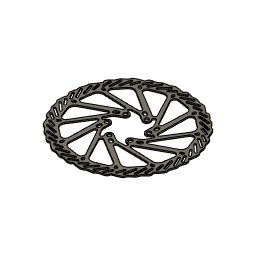
67part (Autodesk Fusion 360 design; units mm, degrees)
Autodesk Fusion 360 part; units mm, degrees
(part 1 of 2)
sketch "Sketch1" plane through (0, 0, 0) normal (0, 1, 0) x (1, 0, 0)
  circle A0 centre (0, 0) radius 80
  circle A1 centre (0, 0) radius 21.9
  dimension "d1" = 160
  dimension "d2" = 43.8
  constraint coincident A0.centre A1.centre
  constraint concentric A0 A1
  measures "d1" diameter of A0
  measures "d2" diameter of A1
sketch "Sketch2" plane through (0, 0, 0) normal (0, 1, 0) x (1, 0, 0)
  spline S0 degree 3 poles (-63.4968, -44.9071) (-64.7262, -42.3768) (-65.0842, -41.971) (-67.4116, -40.491) knots 0 0 0 0 1 1 1 1
  spline S1 degree 3 poles (-67.4116, -40.491) (-69.3332, -39.2736) (-69.9539, -38.6649) (-70.3239, -37.6862) knots 0 0 0 0 1 1 1 1
  spline S2 degree 3 poles (-70.3239, -37.6862) (-70.5984, -36.9224) (-71.5174, -33.3417) (-71.5174, -32.9956) knots 0 0 0 0 1 1 1 1
  spline S3 degree 3 poles (-71.5174, -32.9956) (-71.5174, -32.3869) (-72.1619, -31.1576) (-72.89, -30.3579) knots 0 0 0 0 1 1 1 1
  spline S4 degree 3 poles (-72.89, -30.3579) (-73.7613, -29.4269) (-74.1909, -28.7227) (-74.4416, -27.8873) knots 0 0 0 0 1 1 1 1
  spline S5 degree 3 poles (-74.4416, -27.8873) (-74.6325, -27.2547) (-75.0025, -24.8437) (-75.2174, -22.8625) knots 0 0 0 0 1 1 1 1
  spline S6 degree 3 poles (-75.2174, -22.8625) (-75.3725, -21.4541) (-75.5754, -20.917) (-76.3154, -19.9144) knots 0 0 0 0 1 1 1 1
  spline S7 degree 3 poles (-76.3154, -19.9144) (-77.2464, -18.6851) (-77.4254, -18.1122) (-77.4015, -16.5128) knots 0 0 0 0 1 1 1 1
  spline S8 degree 3 poles (-77.4015, -16.5128) (-77.3777, -14.818) (-77.1986, -11.2254) (-76.9361, -7.2032) knots 0 0 0 0 1 1 1 1
  spline S9 degree 3 poles (-76.9361, -7.2032) (-76.7809, -4.8639) (-76.769, -4.0165) (-76.8645, -3.5271) knots 0 0 0 0 1 1 1 1
  spline S10 degree 3 poles (-76.8645, -3.5271) (-76.9361, -3.181) (-77.497, -1.892) (-78.1057, -0.6626) knots 0 0 0 0 1 1 1 1
  line L0 (-78.1057, -0.6626) -> (-79.2157, 1.5574)
  line L1 (-79.2157, 1.5574) -> (-79.1919, 2.7628)
  spline S11 degree 3 poles (-79.1919, 2.7628) (-79.1799, 4.0041) (-78.9293, 5.0903) (-77.9625, 8.1815) knots 0 0 0 0 1 1 1 1
  line L2 (-77.9625, 8.1815) -> (-77.5686, 9.4109)
  line L3 (-77.5686, 9.4109) -> (-77.7954, 10.4492)
  spline S12 degree 3 poles (-77.7954, 10.4492) (-77.9386, 11.0818) (-78.0222, 11.9412) (-78.0222, 12.6692) knots 0 0 0 0 1 1 1 1
  spline S13 degree 3 poles (-78.0222, 12.6692) (-78.0222, 14.0537) (-77.7357, 15.0444) (-76.4945, 17.9208) knots 0 0 0 0 1 1 1 1
  spline S14 degree 3 poles (-76.4945, 17.9208) (-75.6351, 19.926) (-75.5516, 20.3318) (-75.7306, 21.7759) knots 0 0 0 0 1 1 1 1
  spline S15 degree 3 poles (-75.7306, 21.7759) (-75.9454, 23.5662) (-75.838, 23.8527) (-73.4271, 27.6959) knots 0 0 0 0 1 1 1 1
  spline S16 degree 3 poles (-73.4271, 27.6959) (-72.3051, 29.4743) (-70.9684, 31.5749) (-70.4432, 32.3626) knots 0 0 0 0 1 1 1 1
  spline S17 degree 3 poles (-70.4432, 32.3626) (-69.011, 34.5349) (-68.4858, 35.4062) (-68.2352, 36.0029) knots 0 0 0 0 1 1 1 1
  spline S18 degree 3 poles (-68.2352, 36.0029) (-68.0681, 36.4207) (-67.9845, 37.1368) (-67.8771, 39.13) knots 0 0 0 0 1 1 1 1
  spline S19 degree 3 poles (-67.8771, 39.13) (-67.7458, 41.7081) (-67.7339, 41.72) (-67.34, 42.5077) knots 0 0 0 0 1 1 1 1
  spline S20 degree 3 poles (-67.34, 42.5077) (-67.0058, 43.1522) (-66.5284, 43.7132) (-64.8216, 45.42) knots 0 0 0 0 1 1 1 1
  spline S21 degree 3 poles (-20.3623, 43.2597) (15.6024, 24.417) (-7.9458, 24.9808) (-14.8839, 23.5424) knots 0 0 0 0 1 1 1 1
  spline S22 degree 3 poles (-14.8839, 23.5424) (-16.6504, 23.1724) (-18.3213, 22.8143) (-18.5839, 22.7427) knots 0 0 0 0 1 1 1 1
  spline S23 degree 3 poles (-18.5839, 22.7427) (-20.0042, 22.3369) (-20.78, 20.9524) (-20.2549, 19.735) knots 0 0 0 0 1 1 1 1
  spline S24 degree 3 poles (-20.2549, 19.735) (-19.7894, 18.6608) (-19.2523, 18.3863) (-17.0562, 18.0521) knots 0 0 0 0 1 1 1 1
  spline S25 degree 3 poles (-17.0562, 18.0521) (-16.2446, 17.9327) (-15.6478, 17.7656) (-15.1226, 17.515) knots 0 0 0 0 1 1 1 1
  spline S26 degree 3 poles (-15.1226, 17.515) (-12.3775, 16.1544) (-11.7091, 12.3947) (-13.8097, 10.0076) knots 0 0 0 0 1 1 1 1
  spline S27 degree 3 poles (-13.8097, 10.0076) (-14.5617, 9.1602) (-14.8004, 9.0289) (-17.9275, 7.6683) knots 0 0 0 0 1 1 1 1
  spline S28 degree 3 poles (-17.9275, 7.6683) (-20.7203, 6.4509) (-21.7945, 5.9377) (-22.4032, 5.5199) knots 0 0 0 0 1 1 1 1
  spline S29 degree 3 poles (-22.4032, 5.5199) (-23.0835, 5.0664) (-23.9906, 4.1951) (-24.5516, 3.479) knots 0 0 0 0 1 1 1 1
  spline S30 degree 3 poles (-24.5516, 3.479) (-25.0648, 2.8225) (-25.7332, 1.6767) (-25.6616, 1.5932) knots 0 0 0 0 1 1 1 1
  spline S31 degree 3 poles (-25.6616, 1.5932) (-25.6377, 1.5693) (-25.7213, 1.4141) (-25.8287, 1.2471) knots 0 0 0 0 1 1 1 1
  spline S32 degree 3 poles (-25.8287, 1.2471) (-26.0316, 0.9487) (-27.4996, -3.3839) (-27.9054, -4.8519) knots 0 0 0 0 1 1 1 1
  spline S33 degree 3 poles (-27.9054, -4.8519) (-28.0248, -5.2577) (-28.168, -5.6277) (-28.2396, -5.6755) knots 0 0 0 0 1 1 1 1
  spline S34 degree 3 poles (-28.2396, -5.6755) (-28.3232, -5.7232) (-28.3113, -5.8545) (-28.2038, -6.0455) knots 0 0 0 0 1 1 1 1
  spline S35 degree 3 poles (-28.2038, -6.0455) (-28.1203, -6.2126) (-28.0606, -6.5587) (-28.0964, -6.8332) knots 0 0 0 0 1 1 1 1
  spline S36 degree 3 poles (-28.0964, -6.8332) (-28.1203, -7.1674) (-28.0964, -7.3226) (-27.989, -7.3226) knots 0 0 0 0 1 1 1 1
  spline S37 degree 3 poles (-27.989, -7.3226) (-27.9054, -7.3226) (-27.7861, -7.418) (-27.7264, -7.5493) knots 0 0 0 0 1 1 1 1
  spline S38 degree 3 poles (-27.7264, -7.5493) (-27.5355, -7.8835) (-26.4732, -8.3967) (-25.948, -8.3967) knots 0 0 0 0 1 1 1 1
  spline S39 degree 3 poles (-25.948, -8.3967) (-24.9216, -8.3967) (-24.4681, -8.0984) (-23.4655, -6.7735) knots 0 0 0 0 1 1 1 1
  spline S40 degree 3 poles (-23.4655, -6.7735) (-22.6181, -5.6516) (-21.8781, -4.9832) (-21.0545, -4.6013) knots 0 0 0 0 1 1 1 1
  spline S41 degree 3 poles (-21.0545, -4.6013) (-20.4578, -4.3148) (-20.231, -4.279) (-19.121, -4.279) knots 0 0 0 0 1 1 1 1
  spline S42 degree 3 poles (-19.121, -4.279) (-17.9394, -4.279) (-17.8081, -4.3029) (-17.0681, -4.6729) knots 0 0 0 0 1 1 1 1
  spline S43 degree 3 poles (-17.0681, -4.6729) (-16.161, -5.1145) (-15.242, -6.0335) (-14.8362, -6.8929) knots 0 0 0 0 1 1 1 1
  spline S44 degree 3 poles (-14.8362, -6.8929) (-14.2872, -8.0745) (-14.2752, -8.7548) (-14.693, -12.1564) knots 0 0 0 0 1 1 1 1
  line L4 (-15.1107, -13.3977) -> (-15.0391, -12.6099)
  line L5 (-15.0391, -12.6099) -> (-15.4091, -12.4787)
  spline S45 degree 3 poles (-15.4091, -12.4787) (-15.612, -12.407) (-15.7791, -12.2638) (-15.7791, -12.1683) knots 0 0 0 0 1 1 1 1
  spline S46 degree 3 poles (-15.7791, -12.1683) (-15.7791, -12.049) (-15.7075, -12.0132) (-15.5762, -12.0609) knots 0 0 0 0 1 1 1 1
  spline S47 degree 3 poles (-15.5762, -12.0609) (-15.4449, -12.1087) (-15.4091, -12.0967) (-15.4688, -12.0012) knots 0 0 0 0 1 1 1 1
  spline S48 degree 3 poles (-15.4688, -12.0012) (-15.5165, -11.9177) (-15.4926, -11.858) (-15.433, -11.858) knots 0 0 0 0 1 1 1 1
  spline S49 degree 3 poles (-15.433, -11.858) (-15.3613, -11.858) (-15.3017, -11.8103) (-15.3017, -11.7387) knots 0 0 0 0 1 1 1 1
  spline S50 degree 3 poles (-15.3017, -11.7387) (-15.3017, -11.679) (-15.4091, -11.6193) (-15.5284, -11.6193) knots 0 0 0 0 1 1 1 1
  spline S51 degree 3 poles (-15.5284, -11.6193) (-15.7313, -11.6193) (-15.7433, -11.5716) (-15.6597, -11.2493) knots 0 0 0 0 1 1 1 1
  spline S52 degree 3 poles (-15.6597, -11.2493) (-15.6001, -11.0345) (-15.5762, -10.8196) (-15.612, -10.7719) knots 0 0 0 0 1 1 1 1
  spline S53 degree 3 poles (-15.612, -10.7719) (-15.6478, -10.7122) (-15.6001, -10.6645) (-15.5046, -10.6645) knots 0 0 0 0 1 1 1 1
  spline S54 degree 3 poles (-15.5046, -10.6645) (-15.3255, -10.6645) (-15.1226, -10.9867) (-15.1704, -11.1777) knots 0 0 0 0 1 1 1 1
  spline S55 degree 3 poles (-15.1704, -11.1777) (-15.1823, -11.2374) (-15.1346, -11.2612) (-15.063, -11.2374) knots 0 0 0 0 1 1 1 1
  spline S56 degree 3 poles (-15.063, -11.2374) (-14.9794, -11.2135) (-14.9317, -11.1538) (-14.9436, -11.0941) knots 0 0 0 0 1 1 1 1
  spline S57 degree 3 poles (-14.9436, -11.0941) (-14.9555, -11.0345) (-14.9078, -10.9509) (-14.8362, -10.9032) knots 0 0 0 0 1 1 1 1
  spline S58 degree 3 poles (-14.8362, -10.9032) (-14.5975, -10.76) (-14.8123, -10.4496) (-15.0988, -10.5213) knots 0 0 0 0 1 1 1 1
  line L6 (-15.0988, -10.5213) -> (-15.3613, -10.5809)
  line L7 (-15.3613, -10.5809) -> (-15.1226, -10.3183)
  spline S59 degree 3 poles (-15.1226, -10.3183) (-14.9317, -10.0916) (-14.8839, -9.8648) (-14.872, -9.0055) knots 0 0 0 0 1 1 1 1
  spline S60 degree 3 poles (-14.872, -9.0055) (-14.8601, -8.4445) (-14.8959, -7.9313) (-14.9317, -7.8597) knots 0 0 0 0 1 1 1 1
  spline S61 degree 3 poles (-14.9317, -7.8597) (-14.9794, -7.8) (-15.1226, -7.4777) (-15.242, -7.1435) knots 0 0 0 0 1 1 1 1
  spline S62 degree 3 poles (-15.242, -7.1435) (-15.3852, -6.7258) (-15.6717, -6.3319) (-16.1849, -5.8306) knots 0 0 0 0 1 1 1 1
  spline S63 degree 3 poles (-16.1849, -5.8306) (-16.8175, -5.1981) (-17.0323, -5.0668) (-17.8081, -4.84) knots 0 0 0 0 1 1 1 1
  spline S64 degree 3 poles (-17.8081, -4.84) (-18.7629, -4.5536) (-19.8371, -4.4939) (-19.8371, -4.7087) knots 0 0 0 0 1 1 1 1
  spline S65 degree 3 poles (-19.8371, -4.7087) (-19.8371, -4.7923) (-19.7297, -4.8161) (-19.5507, -4.7684) knots 0 0 0 0 1 1 1 1
  spline S66 degree 3 poles (-19.5507, -4.7684) (-19.3955, -4.7326) (-19.1449, -4.7445) (-18.9897, -4.7923) knots 0 0 0 0 1 1 1 1
  spline S67 degree 3 poles (-18.9897, -4.7923) (-18.7629, -4.8758) (-18.8226, -4.9116) (-19.3716, -5.031) knots 0 0 0 0 1 1 1 1
  spline S68 degree 3 poles (-19.3716, -5.031) (-19.7297, -5.1026) (-20.1236, -5.1981) (-20.2429, -5.2458) knots 0 0 0 0 1 1 1 1
  spline S69 degree 3 poles (-20.2429, -5.2458) (-20.41, -5.3055) (-20.4458, -5.2935) (-20.3861, -5.1861) knots 0 0 0 0 1 1 1 1
  spline S70 degree 3 poles (-20.3861, -5.1861) (-20.3145, -5.0906) (-20.3981, -5.0668) (-20.6965, -5.1145) knots 0 0 0 0 1 1 1 1
  line L8 (-20.6965, -5.1145) -> (-21.0903, -5.1742)
  line L9 (-21.0903, -5.1742) -> (-20.792, -4.9952)
  spline S71 degree 3 poles (-20.792, -4.9952) (-20.41, -4.7803) (-20.6249, -4.7684) (-21.0307, -4.9832) knots 0 0 0 0 1 1 1 1
  line L10 (-21.0307, -4.9832) -> (-21.3171, -5.1503)
  line L11 (-21.3171, -5.1503) -> (-20.8516, -5.2816)
  spline S72 degree 3 poles (-20.8516, -5.2816) (-20.601, -5.3532) (-20.2549, -5.3771) (-20.0878, -5.3413) knots 0 0 0 0 1 1 1 1
  spline S73 degree 3 poles (-20.0878, -5.3413) (-19.8252, -5.2935) (-19.8132, -5.2935) (-19.9923, -5.4129) knots 0 0 0 0 1 1 1 1
  spline S74 degree 3 poles (-19.9923, -5.4129) (-20.0997, -5.4845) (-20.3981, -5.5681) (-20.6487, -5.5919) knots 0 0 0 0 1 1 1 1
  spline S75 degree 3 poles (-20.6487, -5.5919) (-20.8874, -5.6039) (-21.1023, -5.6397) (-21.1142, -5.6516) knots 0 0 0 0 1 1 1 1
  spline S76 degree 3 poles (-21.1142, -5.6516) (-21.1381, -5.6635) (-21.1978, -5.6874) (-21.2574, -5.6993) knots 0 0 0 0 1 1 1 1
  spline S77 degree 3 poles (-21.2574, -5.6993) (-21.3171, -5.6993) (-21.4126, -5.7471) (-21.4603, -5.7948) knots 0 0 0 0 1 1 1 1
  spline S78 degree 3 poles (-21.4603, -5.7948) (-21.5797, -5.9261) (-20.6249, -5.8187) (-20.1355, -5.6516) knots 0 0 0 0 1 1 1 1
  spline S79 degree 3 poles (-20.1355, -5.6516) (-19.9087, -5.58) (-19.67, -5.4368) (-19.6223, -5.3413) knots 0 0 0 0 1 1 1 1
  spline S80 degree 3 poles (-19.6223, -5.3413) (-19.5626, -5.2219) (-19.4433, -5.1981) (-19.3, -5.2458) knots 0 0 0 0 1 1 1 1
  spline S81 degree 3 poles (-19.3, -5.2458) (-19.0852, -5.3294) (-19.0852, -5.3413) (-19.312, -5.4368) knots 0 0 0 0 1 1 1 1
  spline S82 degree 3 poles (-19.312, -5.4368) (-19.4552, -5.4964) (-19.3358, -5.5203) (-18.9658, -5.4726) knots 0 0 0 0 1 1 1 1
  spline S83 degree 3 poles (-18.9658, -5.4726) (-18.572, -5.4368) (-18.4168, -5.4606) (-18.4765, -5.5442) knots 0 0 0 0 1 1 1 1
  spline S84 degree 3 poles (-18.4765, -5.5442) (-18.5242, -5.6277) (-18.4645, -5.6516) (-18.2975, -5.5919) knots 0 0 0 0 1 1 1 1
  spline S85 degree 3 poles (-18.2975, -5.5919) (-18.1662, -5.5561) (-17.9513, -5.5681) (-17.8439, -5.6397) knots 0 0 0 0 1 1 1 1
  spline S86 degree 3 poles (-17.8439, -5.6397) (-17.7126, -5.7113) (-17.6887, -5.771) (-17.7842, -5.771) knots 0 0 0 0 1 1 1 1
  spline S87 degree 3 poles (-17.7842, -5.771) (-17.8678, -5.771) (-17.9036, -5.8306) (-17.8678, -5.9023) knots 0 0 0 0 1 1 1 1
  spline S88 degree 3 poles (-17.8678, -5.9023) (-17.82, -5.9739) (-17.7007, -5.9977) (-17.5933, -5.95) knots 0 0 0 0 1 1 1 1
  spline S89 degree 3 poles (-17.5933, -5.95) (-17.4858, -5.9142) (-17.4381, -5.9142) (-17.4739, -5.9619) knots 0 0 0 0 1 1 1 1
  spline S90 degree 3 poles (-17.4739, -5.9619) (-17.5217, -6.0097) (-17.3784, -6.2603) (-17.1636, -6.5348) knots 0 0 0 0 1 1 1 1
  spline S91 degree 3 poles (-17.1636, -6.5348) (-16.71, -7.0839) (-16.4952, -7.4777) (-16.4952, -7.7045) knots 0 0 0 0 1 1 1 1
  spline S92 degree 3 poles (-16.4952, -7.7045) (-16.4952, -7.788) (-16.6265, -7.6448) (-16.7697, -7.3822) knots 0 0 0 0 1 1 1 1
  spline S93 degree 3 poles (-16.7697, -7.3822) (-17.3546, -6.3558) (-17.9633, -5.9261) (-19.0136, -5.8068) knots 0 0 0 0 1 1 1 1
  spline S94 degree 3 poles (-19.0136, -5.8068) (-20.9829, -5.58) (-22.5106, -7.8239) (-21.6155, -9.6261) knots 0 0 0 0 1 1 1 1
  spline S95 degree 3 poles (-21.6155, -9.6261) (-21.3052, -10.2348) (-20.5532, -10.9867) (-20.1355, -11.0941) knots 0 0 0 0 1 1 1 1
  spline S96 degree 3 poles (-20.1355, -11.0941) (-19.6581, -11.2135) (-17.8916, -11.0822) (-17.832, -10.9271) knots 0 0 0 0 1 1 1 1
  spline S97 degree 3 poles (-17.832, -10.9271) (-17.8081, -10.8435) (-17.6768, -10.7838) (-17.5336, -10.7838) knots 0 0 0 0 1 1 1 1
  spline S98 degree 3 poles (-17.5336, -10.7838) (-17.3665, -10.7838) (-17.5575, -10.9271) (-18.0229, -11.1419) knots 0 0 0 0 1 1 1 1
  spline S99 degree 3 poles (-18.0229, -11.1419) (-19.312, -11.7506) (-20.5532, -11.6193) (-21.4603, -10.76) knots 0 0 0 0 1 1 1 1
  spline S100 degree 3 poles (-21.4603, -10.76) (-21.6871, -10.5451) (-21.8661, -10.4496) (-21.9139, -10.5332) knots 0 0 0 0 1 1 1 1
  spline S101 degree 3 poles (-21.9139, -10.5332) (-21.9616, -10.5929) (-21.8781, -10.7122) (-21.7468, -10.7838) knots 0 0 0 0 1 1 1 1
  spline S102 degree 3 poles (-21.7468, -10.7838) (-21.4365, -10.9509) (-21.4365, -11.1419) (-21.7468, -11.1419) knots 0 0 0 0 1 1 1 1
  spline S103 degree 3 poles (-21.7468, -11.1419) (-21.8781, -11.1419) (-21.9855, -11.0941) (-21.9855, -11.0464) knots 0 0 0 0 1 1 1 1
  spline S104 degree 3 poles (-21.9855, -11.0464) (-21.9855, -10.9987) (-22.1168, -10.939) (-22.2958, -10.9271) knots 0 0 0 0 1 1 1 1
  spline S105 degree 3 poles (-22.2958, -10.9271) (-22.4868, -10.9151) (-22.5703, -10.9509) (-22.5106, -11.0345) knots 0 0 0 0 1 1 1 1
  spline S106 degree 3 poles (-22.5106, -11.0345) (-22.4629, -11.13) (-22.5226, -11.1419) (-22.7135, -11.0822) knots 0 0 0 0 1 1 1 1
  spline S107 degree 3 poles (-22.7135, -11.0822) (-22.8687, -11.0345) (-23.0119, -10.939) (-23.0358, -10.8912) knots 0 0 0 0 1 1 1 1
  spline S108 degree 3 poles (-23.0358, -10.8912) (-23.0955, -10.748) (-23.4177, -10.76) (-23.4177, -10.9032) knots 0 0 0 0 1 1 1 1
  spline S109 degree 3 poles (-23.4177, -10.9032) (-23.4177, -10.9748) (-23.3342, -11.0225) (-23.2268, -11.0225) knots 0 0 0 0 1 1 1 1
  spline S110 degree 3 poles (-23.2268, -11.0225) (-23.0835, -11.0225) (-23.0477, -11.1061) (-23.0835, -11.309) knots 0 0 0 0 1 1 1 1
  spline S111 degree 3 poles (-23.0835, -11.309) (-23.1432, -11.5954) (-23.1313, -11.6074) (-22.809, -11.4283) knots 0 0 0 0 1 1 1 1
  spline S112 degree 3 poles (-22.809, -11.4283) (-22.63, -11.3448) (-22.2958, -11.2732) (-22.081, -11.2732) knots 0 0 0 0 1 1 1 1
  spline S113 degree 3 poles (-22.081, -11.2732) (-21.6871, -11.2971) (-21.6871, -11.2971) (-22.0332, -11.3448) knots 0 0 0 0 1 1 1 1
  spline S114 degree 3 poles (-22.0332, -11.3448) (-22.2958, -11.3925) (-22.3436, -11.4283) (-22.2123, -11.5119) knots 0 0 0 0 1 1 1 1
  spline S115 degree 3 poles (-22.2123, -11.5119) (-22.081, -11.5954) (-22.1048, -11.6193) (-22.3197, -11.6193) knots 0 0 0 0 1 1 1 1
  spline S116 degree 3 poles (-22.3197, -11.6193) (-22.4748, -11.6193) (-22.5584, -11.667) (-22.5226, -11.7387) knots 0 0 0 0 1 1 1 1
  spline S117 degree 3 poles (-22.5226, -11.7387) (-22.4868, -11.8103) (-22.5106, -11.858) (-22.5823, -11.858) knots 0 0 0 0 1 1 1 1
  spline S118 degree 3 poles (-22.5823, -11.858) (-22.6539, -11.858) (-22.6777, -11.9177) (-22.6419, -11.9774) knots 0 0 0 0 1 1 1 1
  spline S119 degree 3 poles (-22.6419, -11.9774) (-22.6061, -12.049) (-22.451, -12.0967) (-22.3077, -12.0967) knots 0 0 0 0 1 1 1 1
  spline S120 degree 3 poles (-22.3077, -12.0967) (-22.069, -12.1087) (-22.069, -12.1206) (-22.26, -12.228) knots 0 0 0 0 1 1 1 1
  spline S121 degree 3 poles (-22.26, -12.228) (-22.3674, -12.2877) (-22.5226, -12.3116) (-22.5942, -12.2638) knots 0 0 0 0 1 1 1 1
  spline S122 degree 3 poles (-22.5942, -12.2638) (-22.6777, -12.2161) (-22.7135, -12.2519) (-22.6777, -12.3474) knots 0 0 0 0 1 1 1 1
  spline S123 degree 3 poles (-22.6777, -12.3474) (-22.6061, -12.5264) (-22.2123, -12.5025) (-22.0929, -12.3116) knots 0 0 0 0 1 1 1 1
  spline S124 degree 3 poles (-22.0929, -12.3116) (-22.0452, -12.2399) (-21.9497, -12.228) (-21.8661, -12.2758) knots 0 0 0 0 1 1 1 1
  spline S125 degree 3 poles (-21.8661, -12.2758) (-21.6513, -12.407) (-22.451, -12.8128) (-22.7016, -12.6935) knots 0 0 0 0 1 1 1 1
  spline S126 degree 3 poles (-22.7016, -12.6935) (-22.7971, -12.6458) (-23.0597, -12.5145) (-23.2626, -12.407) knots 0 0 0 0 1 1 1 1
  spline S127 degree 3 poles (-23.2626, -12.407) (-23.4774, -12.2996) (-23.6564, -12.2519) (-23.6564, -12.3116) knots 0 0 0 0 1 1 1 1
  spline S128 degree 3 poles (-23.6564, -12.3116) (-23.6564, -12.4428) (-22.0571, -13.2903) (-21.8184, -13.2903) knots 0 0 0 0 1 1 1 1
  spline S129 degree 3 poles (-21.8184, -13.2903) (-21.7348, -13.2903) (-21.5558, -13.3977) (-21.4126, -13.529) knots 0 0 0 0 1 1 1 1
  spline S130 degree 3 poles (-21.4126, -13.529) (-21.1739, -13.7557) (-21.15, -13.7557) (-21.15, -13.5648) knots 0 0 0 0 1 1 1 1
  spline S131 degree 3 poles (-21.15, -13.5648) (-21.15, -13.3977) (-21.1142, -13.4216) (-20.9949, -13.6483) knots 0 0 0 0 1 1 1 1
  spline S132 degree 3 poles (-20.9949, -13.6483) (-20.8636, -13.887) (-20.8636, -13.9586) (-20.9949, -13.9825) knots 0 0 0 0 1 1 1 1
  spline S133 degree 3 poles (-20.9949, -13.9825) (-21.0784, -14.0064) (-21.15, -14.0661) (-21.15, -14.1138) knots 0 0 0 0 1 1 1 1
  spline S134 degree 3 poles (-21.15, -14.1138) (-21.15, -14.1615) (-20.8039, -14.1735) (-20.3861, -14.1496) knots 0 0 0 0 1 1 1 1
  spline S135 degree 3 poles (-20.3861, -14.1496) (-19.5984, -14.1019) (-19.2642, -14.2212) (-18.7033, -14.7822) knots 0 0 0 0 1 1 1 1
  spline S136 degree 3 poles (-18.7033, -14.7822) (-18.4526, -15.0209) (-18.0945, -15.9757) (-18.2975, -15.8444) knots 0 0 0 0 1 1 1 1
  spline S137 degree 3 poles (-18.2975, -15.8444) (-18.3571, -15.8086) (-18.4049, -15.7131) (-18.4049, -15.6296) knots 0 0 0 0 1 1 1 1
  spline S138 degree 3 poles (-18.4049, -15.6296) (-18.4049, -15.1522) (-19.6939, -14.2451) (-20.3742, -14.2451) knots 0 0 0 0 1 1 1 1
  spline S139 degree 3 poles (-20.3742, -14.2451) (-20.9352, -14.2451) (-21.6394, -14.7464) (-21.9616, -15.379) knots 0 0 0 0 1 1 1 1
  spline S140 degree 3 poles (-23.8235, -17.1335) (-23.7281, -16.9902) (-23.6684, -16.8231) (-23.7042, -16.7635) knots 0 0 0 0 1 1 1 1
  spline S141 degree 3 poles (-23.7042, -16.7635) (-23.74, -16.7038) (-23.6564, -16.6322) (-23.5252, -16.5964) knots 0 0 0 0 1 1 1 1
  spline S142 degree 3 poles (-23.5252, -16.5964) (-23.2148, -16.5128) (-23.2626, -16.107) (-23.5968, -16.0593) knots 0 0 0 0 1 1 1 1
  spline S143 degree 3 poles (-23.5968, -16.0593) (-23.7997, -16.0235) (-23.7997, -16.0473) (-23.6564, -16.1428) knots 0 0 0 0 1 1 1 1
  spline S144 degree 3 poles (-23.6564, -16.1428) (-23.5252, -16.2383) (-23.6206, -16.2741) (-24.0384, -16.2741) knots 0 0 0 0 1 1 1 1
  spline S145 degree 3 poles (-24.0384, -16.2741) (-24.5755, -16.2741) (-24.7664, -16.1428) (-24.4919, -15.9757) knots 0 0 0 0 1 1 1 1
  spline S146 degree 3 poles (-24.4919, -15.9757) (-24.4322, -15.9399) (-24.4203, -15.8206) (-24.4561, -15.7251) knots 0 0 0 0 1 1 1 1
  spline S147 degree 3 poles (-24.4561, -15.7251) (-24.5039, -15.5819) (-24.4561, -15.5461) (-24.2413, -15.5819) knots 0 0 0 0 1 1 1 1
  spline S148 degree 3 poles (-24.2413, -15.5819) (-24.0264, -15.6057) (-23.9668, -15.5699) (-23.9906, -15.4148) knots 0 0 0 0 1 1 1 1
  spline S149 degree 3 poles (-23.9906, -15.4148) (-24.0264, -15.188) (-23.8355, -15.1164) (-23.7161, -15.3073) knots 0 0 0 0 1 1 1 1
  spline S150 degree 3 poles (-23.7161, -15.3073) (-23.6803, -15.367) (-23.3819, -15.3909) (-23.0477, -15.367) knots 0 0 0 0 1 1 1 1
  spline S151 degree 3 poles (-23.0477, -15.367) (-22.5823, -15.3193) (-22.451, -15.3432) (-22.4868, -15.4625) knots 0 0 0 0 1 1 1 1
  spline S152 degree 3 poles (-22.4868, -15.4625) (-22.5226, -15.5461) (-22.6539, -15.6177) (-22.7852, -15.6177) knots 0 0 0 0 1 1 1 1
  spline S153 degree 3 poles (-22.7852, -15.6177) (-22.9284, -15.6177) (-23.0835, -15.6535) (-23.1313, -15.7131) knots 0 0 0 0 1 1 1 1
  spline S154 degree 3 poles (-23.1313, -15.7131) (-23.179, -15.7609) (-23.1194, -15.7967) (-23, -15.7967) knots 0 0 0 0 1 1 1 1
  spline S155 degree 3 poles (-23, -15.7967) (-22.8806, -15.7967) (-22.7135, -15.8922) (-22.63, -16.0115) knots 0 0 0 0 1 1 1 1
  spline S156 degree 3 poles (-22.63, -16.0115) (-22.4748, -16.2025) (-22.4748, -16.2025) (-22.4629, -15.9757) knots 0 0 0 0 1 1 1 1
  spline S157 degree 3 poles (-22.4629, -15.9757) (-22.4629, -15.8444) (-22.3555, -15.5819) (-22.2242, -15.379) knots 0 0 0 0 1 1 1 1
  spline S158 degree 3 poles (-22.2242, -15.379) (-21.9258, -14.9373) (-21.9258, -14.9015) (-22.2123, -14.8777) knots 0 0 0 0 1 1 1 1
  spline S159 degree 3 poles (-22.2123, -14.8777) (-22.3913, -14.8657) (-22.4271, -14.9135) (-22.3794, -15.0567) knots 0 0 0 0 1 1 1 1
  spline S160 degree 3 poles (-22.3794, -15.0567) (-22.3077, -15.2477) (-22.3197, -15.2357) (-22.5465, -15.0567) knots 0 0 0 0 1 1 1 1
  spline S161 degree 3 poles (-22.5465, -15.0567) (-22.6777, -14.9373) (-22.8806, -14.8419) (-23.0119, -14.8538) knots 0 0 0 0 1 1 1 1
  spline S162 degree 3 poles (-23.0119, -14.8538) (-23.2268, -14.8538) (-23.2268, -14.8657) (-23, -14.9493) knots 0 0 0 0 1 1 1 1
  spline S163 degree 3 poles (-23, -14.9493) (-22.7613, -15.0448) (-22.7613, -15.0448) (-23.0119, -15.1283) knots 0 0 0 0 1 1 1 1
  spline S164 degree 3 poles (-23.0119, -15.1283) (-23.4894, -15.2715) (-23.8952, -14.997) (-23.8952, -14.5315) knots 0 0 0 0 1 1 1 1
  spline S165 degree 3 poles (-23.8952, -14.5315) (-23.8952, -14.3883) (-23.9787, -14.2451) (-24.0742, -14.1974) knots 0 0 0 0 1 1 1 1
  spline S166 degree 3 poles (-24.0742, -14.1974) (-24.1697, -14.1615) (-24.2532, -14.078) (-24.2532, -14.0064) knots 0 0 0 0 1 1 1 1
  spline S167 degree 3 poles (-24.2532, -14.0064) (-24.2532, -13.8512) (-23.6923, -13.8512) (-23.5968, -14.0064) knots 0 0 0 0 1 1 1 1
  spline S168 degree 3 poles (-23.5968, -14.0064) (-23.549, -14.078) (-23.4655, -14.1019) (-23.4058, -14.0541) knots 0 0 0 0 1 1 1 1
  spline S169 degree 3 poles (-23.4058, -14.0541) (-23.3342, -14.0183) (-23.3461, -13.9109) (-23.4416, -13.7915) knots 0 0 0 0 1 1 1 1
  spline S170 degree 3 poles (-23.4416, -13.7915) (-23.5848, -13.6364) (-23.561, -13.6245) (-23.3342, -13.7557) knots 0 0 0 0 1 1 1 1
  spline S171 degree 3 poles (-23.3342, -13.7557) (-23.1552, -13.8393) (-23.0716, -13.9825) (-23.0955, -14.1615) knots 0 0 0 0 1 1 1 1
  spline S172 degree 3 poles (-23.0955, -14.1615) (-23.1194, -14.3883) (-23.0716, -14.4122) (-22.7255, -14.3883) knots 0 0 0 0 1 1 1 1
  spline S173 degree 3 poles (-22.7255, -14.3883) (-22.439, -14.3525) (-22.3436, -14.3883) (-22.3436, -14.5315) knots 0 0 0 0 1 1 1 1
  spline S174 degree 3 poles (-22.3436, -14.5315) (-22.3436, -14.8061) (-21.8423, -14.7703) (-21.5319, -14.4838) knots 0 0 0 0 1 1 1 1
  spline S175 degree 3 poles (-21.5319, -14.4838) (-21.2574, -14.2212) (-21.1858, -14.0064) (-21.3768, -14.0064) knots 0 0 0 0 1 1 1 1
  spline S176 degree 3 poles (-21.3768, -14.0064) (-21.4365, -14.0064) (-21.5081, -14.0541) (-21.5319, -14.1138) knots 0 0 0 0 1 1 1 1
  spline S177 degree 3 poles (-21.5319, -14.1138) (-21.5797, -14.269) (-22.6181, -13.7438) (-22.6539, -13.5528) knots 0 0 0 0 1 1 1 1
  spline S178 degree 3 poles (-22.6539, -13.5528) (-22.6658, -13.4693) (-22.6539, -13.4574) (-22.63, -13.517) knots 0 0 0 0 1 1 1 1
  spline S179 degree 3 poles (-22.63, -13.517) (-22.5584, -13.6603) (-22.2242, -13.5528) (-22.2242, -13.3977) knots 0 0 0 0 1 1 1 1
  spline S180 degree 3 poles (-22.2242, -13.3977) (-22.2242, -13.338) (-22.2958, -13.2903) (-22.3913, -13.2903) knots 0 0 0 0 1 1 1 1
  spline S181 degree 3 poles (-22.3913, -13.2903) (-22.4748, -13.2903) (-22.6181, -13.2187) (-22.6897, -13.1232) knots 0 0 0 0 1 1 1 1
  spline S182 degree 3 poles (-22.6897, -13.1232) (-22.7971, -12.9919) (-23.1432, -12.8725) (-23.6206, -12.8009) knots 0 0 0 0 1 1 1 1
  spline S183 degree 3 poles (-23.6206, -12.8009) (-23.6684, -12.8009) (-23.7281, -12.8606) (-23.7639, -12.9441) knots 0 0 0 0 1 1 1 1
  spline S184 degree 3 poles (-23.7639, -12.9441) (-23.7877, -13.0277) (-23.7519, -13.0516) (-23.6684, -13.0038) knots 0 0 0 0 1 1 1 1
  spline S185 degree 3 poles (-23.6684, -13.0038) (-23.5968, -12.9561) (-23.5371, -12.9799) (-23.5371, -13.0516) knots 0 0 0 0 1 1 1 1
  spline S186 degree 3 poles (-23.5371, -13.0516) (-23.5371, -13.1232) (-23.4894, -13.159) (-23.4177, -13.1112) knots 0 0 0 0 1 1 1 1
  spline S187 degree 3 poles (-23.4177, -13.1112) (-23.2387, -13.0038) (-22.821, -13.3261) (-22.821, -13.5648) knots 0 0 0 0 1 1 1 1
  spline S188 degree 3 poles (-22.821, -13.5648) (-22.821, -13.8751) (-23.0955, -13.7557) (-23.191, -13.3977) knots 0 0 0 0 1 1 1 1
  spline S189 degree 3 poles (-23.191, -13.3977) (-23.2506, -13.2067) (-23.2745, -13.1828) (-23.2864, -13.3261) knots 0 0 0 0 1 1 1 1
  spline S190 degree 3 poles (-23.2864, -13.3261) (-23.2984, -13.5767) (-23.6087, -13.5886) (-23.7042, -13.338) knots 0 0 0 0 1 1 1 1
  spline S191 degree 3 poles (-23.7042, -13.338) (-23.7639, -13.1828) (-23.8116, -13.1709) (-23.9429, -13.2783) knots 0 0 0 0 1 1 1 1
  spline S192 degree 3 poles (-23.9429, -13.2783) (-24.0742, -13.3857) (-24.1219, -13.3499) (-24.1816, -13.1232) knots 0 0 0 0 1 1 1 1
  spline S193 degree 3 poles (-24.1816, -13.1232) (-24.2174, -12.968) (-24.2174, -12.7532) (-24.1816, -12.6577) knots 0 0 0 0 1 1 1 1
  spline S194 degree 3 poles (-24.1816, -12.6577) (-24.1458, -12.5622) (-24.1697, -12.4428) (-24.2413, -12.3951) knots 0 0 0 0 1 1 1 1
  spline S195 degree 3 poles (-24.2413, -12.3951) (-24.3248, -12.3593) (-24.3726, -12.4309) (-24.3726, -12.5741) knots 0 0 0 0 1 1 1 1
  spline S196 degree 3 poles (-24.3726, -12.5741) (-24.3726, -12.7651) (-24.4322, -12.8128) (-24.5874, -12.7651) knots 0 0 0 0 1 1 1 1
  spline S197 degree 3 poles (-24.5874, -12.7651) (-24.7187, -12.7174) (-24.85, -12.777) (-24.9335, -12.9322) knots 0 0 0 0 1 1 1 1
  spline S198 degree 3 poles (-24.9335, -12.9322) (-25.1245, -13.2187) (-24.9335, -13.3619) (-24.6948, -13.1112) knots 0 0 0 0 1 1 1 1
  spline S199 degree 3 poles (-24.6948, -13.1112) (-24.4561, -12.8845) (-24.4322, -12.8845) (-24.4084, -13.1709) knots 0 0 0 0 1 1 1 1
  spline S200 degree 3 poles (-24.4084, -13.1709) (-24.3964, -13.3022) (-24.4322, -13.4096) (-24.5039, -13.4096) knots 0 0 0 0 1 1 1 1
  spline S201 degree 3 poles (-24.5039, -13.4096) (-24.5635, -13.4096) (-24.6113, -13.4932) (-24.6113, -13.5886) knots 0 0 0 0 1 1 1 1
  spline S202 degree 3 poles (-24.6113, -13.5886) (-24.6113, -13.6841) (-24.6948, -13.7677) (-24.8022, -13.7677) knots 0 0 0 0 1 1 1 1
  spline S203 degree 3 poles (-24.8022, -13.7677) (-24.8977, -13.7677) (-24.9574, -13.8154) (-24.9097, -13.8751) knots 0 0 0 0 1 1 1 1
  spline S204 degree 3 poles (-24.9097, -13.8751) (-24.8739, -13.9348) (-24.8977, -14.0183) (-24.9574, -14.0541) knots 0 0 0 0 1 1 1 1
  spline S205 degree 3 poles (-24.9574, -14.0541) (-25.0171, -14.1019) (-25.1364, -13.9706) (-25.2319, -13.7677) knots 0 0 0 0 1 1 1 1
  spline S206 degree 3 poles (-25.2319, -13.7677) (-25.3155, -13.5767) (-25.4468, -13.4096) (-25.5303, -13.4096) knots 0 0 0 0 1 1 1 1
  spline S207 degree 3 poles (-25.5303, -13.4096) (-25.7093, -13.4096) (-25.578, -13.9109) (-25.3393, -14.0899) knots 0 0 0 0 1 1 1 1
  spline S208 degree 3 poles (-25.3393, -14.0899) (-25.1006, -14.2809) (-24.6113, -14.2928) (-24.6113, -14.1138) knots 0 0 0 0 1 1 1 1
  spline S209 degree 3 poles (-24.6113, -14.1138) (-24.6113, -14.0183) (-24.5516, -14.0183) (-24.4322, -14.1257) knots 0 0 0 0 1 1 1 1
  spline S210 degree 3 poles (-24.4322, -14.1257) (-24.1339, -14.3644) (-24.2293, -14.448) (-24.7306, -14.4241) knots 0 0 0 0 1 1 1 1
  spline S211 degree 3 poles (-24.7306, -14.4241) (-24.9932, -14.4122) (-25.2439, -14.448) (-25.2797, -14.4957) knots 0 0 0 0 1 1 1 1
  spline S212 degree 3 poles (-25.2797, -14.4957) (-25.3155, -14.5554) (-25.2319, -14.6032) (-25.0887, -14.6032) knots 0 0 0 0 1 1 1 1
  spline S213 degree 3 poles (-25.0887, -14.6032) (-24.9455, -14.6032) (-24.8739, -14.6628) (-24.9097, -14.7225) knots 0 0 0 0 1 1 1 1
  spline S214 degree 3 poles (-24.9097, -14.7225) (-24.9574, -14.7941) (-25.041, -14.818) (-25.1006, -14.7822) knots 0 0 0 0 1 1 1 1
  spline S215 degree 3 poles (-25.1006, -14.7822) (-25.1603, -14.7344) (-25.208, -14.7703) (-25.208, -14.8419) knots 0 0 0 0 1 1 1 1
  spline S216 degree 3 poles (-25.208, -14.8419) (-25.208, -15.0328) (-24.8381, -15.1402) (-24.7306, -14.9732) knots 0 0 0 0 1 1 1 1
  spline S217 degree 3 poles (-24.7306, -14.9732) (-24.671, -14.8657) (-24.6232, -14.9135) (-24.5874, -15.1164) knots 0 0 0 0 1 1 1 1
  spline S218 degree 3 poles (-24.5874, -15.1164) (-24.5397, -15.3551) (-24.5755, -15.3909) (-24.7545, -15.3432) knots 0 0 0 0 1 1 1 1
  spline S219 degree 3 poles (-24.7545, -15.3432) (-25.029, -15.2715) (-25.041, -15.5341) (-24.7545, -15.749) knots 0 0 0 0 1 1 1 1
  spline S220 degree 3 poles (-24.7545, -15.749) (-24.6471, -15.8325) (-24.6113, -15.9161) (-24.6829, -15.9161) knots 0 0 0 0 1 1 1 1
  spline S221 degree 3 poles (-24.6829, -15.9161) (-24.8381, -15.9161) (-24.7545, -16.5128) (-24.5993, -16.5128) knots 0 0 0 0 1 1 1 1
  spline S222 degree 3 poles (-24.5993, -16.5128) (-24.3845, -16.5128) (-24.4919, -16.9664) (-24.7187, -17.026) knots 0 0 0 0 1 1 1 1
  spline S223 degree 3 poles (-24.7187, -17.026) (-24.9097, -17.0738) (-24.9574, -16.9902) (-25.0171, -16.3696) knots 0 0 0 0 1 1 1 1
  spline S224 degree 3 poles (-25.0171, -16.3696) (-25.0648, -15.9757) (-25.2797, -15.1402) (-25.5064, -14.4957) knots 0 0 0 0 1 1 1 1
  spline S225 degree 3 poles (-25.5064, -14.4957) (-26.4493, -11.7864) (-27.2013, -10.9748) (-28.8006, -10.9629) knots 0 0 0 0 1 1 1 1
  spline S226 degree 3 poles (-28.8006, -10.9629) (-29.5645, -10.9629) (-29.6361, -10.9867) (-30.4477, -11.5477) knots 0 0 0 0 1 1 1 1
  spline S227 degree 3 poles (-30.4477, -11.5477) (-30.9132, -11.858) (-31.6293, -12.4906) (-32.047, -12.9322) knots 0 0 0 0 1 1 1 1
  spline S228 degree 3 poles (-32.047, -12.9322) (-32.7393, -13.6841) (-33.0854, -14.1854) (-35.0786, -17.3483) knots 0 0 0 0 1 1 1 1
  spline S229 degree 3 poles (-35.0786, -17.3483) (-35.5083, -18.0406) (-36.0931, -18.9476) (-36.3676, -19.3773) knots 0 0 0 0 1 1 1 1
  spline S230 degree 3 poles (-36.3676, -19.3773) (-37.1196, -20.5351) (-39.256, -23.9963) (-40.3063, -25.7628) knots 0 0 0 0 1 1 1 1
  spline S231 degree 3 poles (-40.3063, -25.7628) (-40.8076, -26.6221) (-41.6431, -28.0185) (-42.1563, -28.866) knots 0 0 0 0 1 1 1 1
  spline S232 degree 3 poles (-42.1563, -28.866) (-45.9518, -35.2395) (-47.5511, -38.0323) (-47.933, -38.9991) knots 0 0 0 0 1 1 1 1
  spline S233 degree 3 poles (-47.933, -38.9991) (-48.7566, -41.052) (-48.4463, -43.7255) (-47.1692, -45.6829) knots 0 0 0 0 1 1 1 1
  spline S234 degree 3 poles (-52.1821, -47.4136) (-52.6714, -47.2703) (-53.2324, -47.0913) (-53.4353, -47.0078) knots 0 0 0 0 1 1 1 1
  spline S235 degree 3 poles (-53.4353, -47.0078) (-53.6262, -46.9242) (-54.3782, -46.6497) (-55.1062, -46.3991) knots 0 0 0 0 1 1 1 1
  spline S236 degree 3 poles (-55.1062, -46.3991) (-55.8223, -46.1484) (-57.171, -45.6352) (-58.0781, -45.2652) knots 0 0 0 0 1 1 1 1
  spline S237 degree 3 poles (-58.0781, -45.2652) (-58.9972, -44.8952) (-59.8207, -44.6088) (-59.9043, -44.6446) knots 0 0 0 0 1 1 1 1
  spline S238 degree 3 poles (-59.9043, -44.6446) (-60.3101, -44.7997) (-59.9401, -46.3036) (-59.3672, -46.8049) knots 0 0 0 0 1 1 1 1
  spline S239 degree 3 poles (-59.3672, -46.8049) (-56.4924, -51.4425) (-45.3417, -49.4341) (-52.1821, -47.4136) knots 0 0 0 0 1 1 1 1
  spline S240 degree 3 poles (-52.6475, -41.3265) (-52.4566, -41.1236) (-52.194, -40.7059) (-52.0508, -40.3956) knots 0 0 0 0 1 1 1 1
  spline S241 degree 3 poles (-52.0508, -40.3956) (-51.6688, -39.5481) (-51.2272, -38.3427) (-51.2272, -38.1636) knots 0 0 0 0 1 1 1 1
  spline S242 degree 3 poles (-51.2272, -38.1636) (-51.2272, -38.0801) (-51.3943, -37.8175) (-51.5972, -37.5788) knots 0 0 0 0 1 1 1 1
  spline S243 degree 3 poles (-51.5972, -37.5788) (-51.8956, -37.2446) (-52.0508, -37.1611) (-52.4088, -37.1611) knots 0 0 0 0 1 1 1 1
  spline S244 degree 3 poles (-52.4088, -37.1611) (-52.922, -37.1611) (-54.0201, -37.7698) (-54.8795, -38.5336) knots 0 0 0 0 1 1 1 1
  spline S245 degree 3 poles (-54.8795, -38.5336) (-55.4165, -38.9991) (-55.4523, -39.0588) (-55.5001, -39.751) knots 0 0 0 0 1 1 1 1
  spline S246 degree 3 poles (-55.5001, -39.751) (-55.5598, -40.5865) (-55.3927, -40.9446) (-54.7004, -41.4101) knots 0 0 0 0 1 1 1 1
  spline S247 degree 3 poles (-54.7004, -41.4101) (-54.3782, -41.6249) (-54.1156, -41.6965) (-53.6382, -41.6965) knots 0 0 0 0 1 1 1 1
  spline S248 degree 3 poles (-53.6382, -41.6965) (-53.0772, -41.6965) (-52.9459, -41.6488) (-52.6475, -41.3265) knots 0 0 0 0 1 1 1 1
  spline S249 degree 3 poles (-58.7823, -41.4817) (-58.472, -41.2907) (-58.472, -40.7536) (-58.7943, -40.1091) knots 0 0 0 0 1 1 1 1
  spline S250 degree 3 poles (-58.7943, -40.1091) (-59.0926, -39.4885) (-59.1523, -39.4407) (-60.501, -38.7246) knots 0 0 0 0 1 1 1 1
  spline S251 degree 3 poles (-60.501, -38.7246) (-61.2768, -38.3188) (-61.9929, -37.9369) (-62.0884, -37.8772) knots 0 0 0 0 1 1 1 1
  spline S252 degree 3 poles (-62.0884, -37.8772) (-62.1839, -37.8175) (-62.6136, -37.5788) (-63.0433, -37.352) knots 0 0 0 0 1 1 1 1
  spline S253 degree 3 poles (-63.0433, -37.352) (-63.9384, -36.8865) (-64.762, -36.4091) (-66.4329, -35.4304) knots 0 0 0 0 1 1 1 1
  spline S254 degree 3 poles (-66.4329, -35.4304) (-67.5548, -34.762) (-67.6145, -34.7382) (-67.7697, -34.953) knots 0 0 0 0 1 1 1 1
  spline S255 degree 3 poles (-67.7697, -34.953) (-68.1397, -35.4543) (-67.889, -36.5882) (-67.2684, -37.1969) knots 0 0 0 0 1 1 1 1
  spline S256 degree 3 poles (-67.2684, -37.1969) (-66.2061, -38.2591) (-61.432, -40.8372) (-59.3552, -41.4578) knots 0 0 0 0 1 1 1 1
  spline S257 degree 3 poles (-59.3552, -41.4578) (-58.9494, -41.5891) (-58.9494, -41.5891) (-58.7823, -41.4817) knots 0 0 0 0 1 1 1 1
  spline S258 degree 3 poles (-59.4507, -35.2514) (-58.9017, -34.953) (-59.4388, -33.7595) (-60.3936, -33.1627) knots 0 0 0 0 1 1 1 1
  spline S259 degree 3 poles (-60.3936, -33.1627) (-61.2171, -32.6495) (-64.4397, -30.525) (-64.8097, -30.2385) knots 0 0 0 0 1 1 1 1
  spline S260 degree 3 poles (-64.8097, -30.2385) (-64.9887, -30.1072) (-65.9078, -29.4269) (-66.8626, -28.7227) knots 0 0 0 0 1 1 1 1
  spline S261 degree 3 poles (-66.8626, -28.7227) (-67.8174, -28.0185) (-68.6529, -27.386) (-68.7245, -27.3144) knots 0 0 0 0 1 1 1 1
  spline S262 degree 3 poles (-68.7245, -27.3144) (-68.7961, -27.2547) (-69.0348, -27.0637) (-69.2497, -26.8966) knots 0 0 0 0 1 1 1 1
  spline S263 degree 3 poles (-69.2497, -26.8966) (-69.4645, -26.7295) (-70.0255, -26.2879) (-70.479, -25.9179) knots 0 0 0 0 1 1 1 1
  spline S264 degree 3 poles (-70.479, -25.9179) (-71.398, -25.1421) (-71.6964, -25.0705) (-71.8874, -25.5599) knots 0 0 0 0 1 1 1 1
  spline S265 degree 3 poles (-71.8874, -25.5599) (-72.0664, -25.9895) (-71.7561, -27.2308) (-71.2787, -27.9708) knots 0 0 0 0 1 1 1 1
  spline S266 degree 3 poles (-71.2787, -27.9708) (-70.8132, -28.6989) (-68.8439, -30.155) (-65.3587, -32.3511) knots 0 0 0 0 1 1 1 1
  spline S267 degree 3 poles (-65.3587, -32.3511) (-63.4849, -33.5327) (-60.1788, -35.323) (-59.7849, -35.3588) knots 0 0 0 0 1 1 1 1
  spline S268 degree 3 poles (-59.7849, -35.3588) (-59.7252, -35.3708) (-59.582, -35.3111) (-59.4507, -35.2514) knots 0 0 0 0 1 1 1 1
  spline S269 degree 3 poles (-51.8956, -33.4133) (-51.4062, -33.2104) (-50.165, -32.2556) (-49.234, -31.3963) knots 0 0 0 0 1 1 1 1
  spline S270 degree 3 poles (-49.234, -31.3963) (-48.494, -30.704) (-46.6321, -28.3169) (-45.3431, -26.4192) knots 0 0 0 0 1 1 1 1
  spline S271 degree 3 poles (-45.3431, -26.4192) (-44.9611, -25.8582) (-44.1257, -24.6528) (-43.4692, -23.7337) knots 0 0 0 0 1 1 1 1
  spline S272 degree 3 poles (-43.4692, -23.7337) (-41.4283, -20.8573) (-40.4137, -19.3415) (-38.6831, -16.5725) knots 0 0 0 0 1 1 1 1
  spline S273 degree 3 poles (-38.6831, -16.5725) (-37.9312, -15.3909) (-37.2867, -14.3764) (-37.2389, -14.3048) knots 0 0 0 0 1 1 1 1
  spline S274 degree 3 poles (-37.2389, -14.3048) (-37.0838, -14.1257) (-35.6635, -11.7625) (-34.6012, -9.9245) knots 0 0 0 0 1 1 1 1
  spline S275 degree 3 poles (-34.6012, -9.9245) (-34.076, -9.0174) (-33.5986, -8.2774) (-33.5509, -8.2774) knots 0 0 0 0 1 1 1 1
  spline S276 degree 3 poles (-33.5509, -8.2774) (-33.4912, -8.2774) (-33.4435, -8.2058) (-33.4435, -8.1103) knots 0 0 0 0 1 1 1 1
  spline S277 degree 3 poles (-33.4435, -8.1103) (-33.4435, -8.0268) (-33.169, -7.4777) (-32.8348, -6.8929) knots 0 0 0 0 1 1 1 1
  spline S278 degree 3 poles (-32.8348, -6.8929) (-31.4025, -4.4103) (-29.8748, -1.4742) (-29.5883, -0.6387) knots 0 0 0 0 1 1 1 1
  spline S279 degree 3 poles (-29.5883, -0.6387) (-28.9319, 1.2471) (-28.6932, 3.109) (-29.0035, 4.0519) knots 0 0 0 0 1 1 1 1
  spline S280 degree 3 poles (-29.0035, 4.0519) (-29.4212, 5.329) (-30.4358, 5.9138) (-32.0232, 5.7586) knots 0 0 0 0 1 1 1 1
  spline S281 degree 3 poles (-32.0232, 5.7586) (-34.1119, 5.5438) (-35.1264, 5.1141) (-40.6047, 2.1064) knots 0 0 0 0 1 1 1 1
  spline S282 degree 3 poles (-40.6047, 2.1064) (-41.3566, 1.7006) (-42.8128, 0.9129) (-43.8273, 0.3758) knots 0 0 0 0 1 1 1 1
  spline S283 degree 3 poles (-43.8273, 0.3758) (-46.7992, -1.2116) (-48.8879, -2.3694) (-53.674, -5.1145) knots 0 0 0 0 1 1 1 1
  spline S284 degree 3 poles (-53.674, -5.1145) (-60.2026, -8.8503) (-60.7517, -9.2203) (-61.6468, -10.2945) knots 0 0 0 0 1 1 1 1
  spline S285 degree 3 poles (-61.6468, -10.2945) (-62.172, -10.939) (-62.8284, -12.2877) (-63.0313, -13.1112) knots 0 0 0 0 1 1 1 1
  spline S286 degree 3 poles (-63.0313, -13.1112) (-63.2939, -14.1735) (-63.2104, -15.8206) (-62.8165, -17.3483) knots 0 0 0 0 1 1 1 1
  spline S287 degree 3 poles (-62.8165, -17.3483) (-62.6255, -18.1002) (-62.4107, -18.888) (-62.3391, -19.0789) knots 0 0 0 0 1 1 1 1
  spline S288 degree 3 poles (-62.3391, -19.0789) (-62.2675, -19.2818) (-62.0407, -19.998) (-61.8259, -20.6902) knots 0 0 0 0 1 1 1 1
  spline S289 degree 3 poles (-61.8259, -20.6902) (-61.432, -21.9912) (-60.7159, -24.0202) (-60.2743, -25.0466) knots 0 0 0 0 1 1 1 1
  spline S290 degree 3 poles (-60.2743, -25.0466) (-60.143, -25.3808) (-59.9878, -25.7508) (-59.9401, -25.8821) knots 0 0 0 0 1 1 1 1
  spline S291 degree 3 poles (-59.9401, -25.8821) (-59.8923, -26.0134) (-59.7133, -26.4192) (-59.5462, -26.7773) knots 0 0 0 0 1 1 1 1
  spline S292 degree 3 poles (-59.5462, -26.7773) (-59.3791, -27.1353) (-59.1404, -27.7082) (-59.0091, -28.0305) knots 0 0 0 0 1 1 1 1
  spline S293 degree 3 poles (-59.0091, -28.0305) (-58.4243, -29.5105) (-57.171, -31.7901) (-56.6578, -32.3153) knots 0 0 0 0 1 1 1 1
  spline S294 degree 3 poles (-56.6578, -32.3153) (-56.0611, -32.9121) (-55.1301, -33.4133) (-54.3304, -33.5685) knots 0 0 0 0 1 1 1 1
  spline S295 degree 3 poles (-54.3304, -33.5685) (-53.674, -33.7117) (-52.385, -33.6162) (-51.8956, -33.4133) knots 0 0 0 0 1 1 1 1
  spline S296 degree 3 poles (-63.4133, -26.5863) (-63.1746, -26.276) (-63.1746, -26.276) (-63.4013, -25.8344) knots 0 0 0 0 1 1 1 1
  spline S297 degree 3 poles (-63.4013, -25.8344) (-63.5207, -25.5837) (-63.9504, -25.0944) (-64.3562, -24.7363) knots 0 0 0 0 1 1 1 1
  spline S298 degree 3 poles (-64.3562, -24.7363) (-64.7739, -24.3782) (-65.4303, -23.7934) (-65.8361, -23.4354) knots 0 0 0 0 1 1 1 1
  spline S299 degree 3 poles (-65.8361, -23.4354) (-66.23, -23.0654) (-66.8865, -22.5044) (-67.2803, -22.1821) knots 0 0 0 0 1 1 1 1
  spline S300 degree 3 poles (-67.2803, -22.1821) (-67.6742, -21.8599) (-69.3571, -20.2367) (-71.0161, -18.5776) knots 0 0 0 0 1 1 1 1
  spline S301 degree 3 poles (-71.0161, -18.5776) (-74.1909, -15.4028) (-74.5132, -15.1641) (-74.6922, -15.8683) knots 0 0 0 0 1 1 1 1
  spline S302 degree 3 poles (-74.6922, -15.8683) (-74.8116, -16.3577) (-74.6683, -17.2409) (-74.3342, -18.0047) knots 0 0 0 0 1 1 1 1
  spline S303 degree 3 poles (-74.3342, -18.0047) (-74.0358, -18.6612) (-73.1764, -19.616) (-71.6248, -20.9886) knots 0 0 0 0 1 1 1 1
  spline S304 degree 3 poles (-71.6248, -20.9886) (-69.6197, -22.7789) (-69.011, -23.2921) (-67.8174, -24.2231) knots 0 0 0 0 1 1 1 1
  spline S305 degree 3 poles (-67.8174, -24.2231) (-65.3707, -26.1328) (-64.2487, -26.8966) (-63.8549, -26.8966) knots 0 0 0 0 1 1 1 1
  spline S306 degree 3 poles (-63.8549, -26.8966) (-63.7475, -26.8966) (-63.5446, -26.7534) (-63.4133, -26.5863) knots 0 0 0 0 1 1 1 1
  spline S307 degree 3 poles (-67.4832, -17.1454) (-67.4236, -17.026) (-67.34, -16.7038) (-67.2923, -16.4173) knots 0 0 0 0 1 1 1 1
  spline S308 degree 3 poles (-67.2923, -16.4173) (-67.2087, -15.8206) (-67.4474, -15.2596) (-68.0681, -14.6032) knots 0 0 0 0 1 1 1 1
  spline S309 degree 3 poles (-68.0681, -14.6032) (-69.3929, -13.1948) (-71.2309, -11.0345) (-72.3887, -9.5067) knots 0 0 0 0 1 1 1 1
  spline S310 degree 3 poles (-72.3887, -9.5067) (-72.878, -8.8622) (-73.3554, -8.2655) (-73.4629, -8.1819) knots 0 0 0 0 1 1 1 1
  spline S311 degree 3 poles (-73.4629, -8.1819) (-73.7493, -7.9432) (-74.0358, -8.0506) (-74.2864, -8.5161) knots 0 0 0 0 1 1 1 1
  spline S312 degree 3 poles (-74.2864, -8.5161) (-74.6325, -9.1487) (-74.5132, -10.1393) (-73.9761, -10.939) knots 0 0 0 0 1 1 1 1
  spline S313 degree 3 poles (-73.9761, -10.939) (-73.5464, -11.5716) (-72.4961, -12.9203) (-71.9113, -13.5767) knots 0 0 0 0 1 1 1 1
  spline S314 degree 3 poles (-71.9113, -13.5767) (-68.8319, -17.026) (-67.8294, -17.8257) (-67.4832, -17.1454) knots 0 0 0 0 1 1 1 1
  spline S315 degree 3 poles (-65.0603, -8.2655) (-63.9026, -7.5135) (-63.2581, -6.9526) (-63.0791, -6.5229) knots 0 0 0 0 1 1 1 1
  spline S316 degree 3 poles (-63.0791, -6.5229) (-62.8523, -5.9739) (-62.8762, -5.8664) (-63.2939, -5.4368) knots 0 0 0 0 1 1 1 1
  spline S317 degree 3 poles (-63.2939, -5.4368) (-63.64, -5.0787) (-63.7236, -5.0548) (-64.4636, -5.0548) knots 0 0 0 0 1 1 1 1
  spline S318 degree 3 poles (-64.4636, -5.0548) (-65.5378, -5.0548) (-66.8626, -5.2577) (-67.1848, -5.4726) knots 0 0 0 0 1 1 1 1
  spline S319 degree 3 poles (-67.1848, -5.4726) (-67.889, -5.9381) (-68.1039, -7.1555) (-67.6145, -7.9193) knots 0 0 0 0 1 1 1 1
  spline S320 degree 3 poles (-67.6145, -7.9193) (-67.0058, -8.8861) (-66.1942, -8.9935) (-65.0603, -8.2655) knots 0 0 0 0 1 1 1 1
  spline S321 degree 3 poles (-70.849, -5.5203) (-70.67, -5.3174) (-70.6222, -5.0906) (-70.6222, -4.3865) knots 0 0 0 0 1 1 1 1
  spline S322 degree 3 poles (-70.6222, -4.3865) (-70.6222, -3.8971) (-70.6819, -3.4555) (-70.7416, -3.4078) knots 0 0 0 0 1 1 1 1
  spline S323 degree 3 poles (-70.7416, -3.4078) (-70.9684, -3.2526) (-74.0835, 1.7603) (-74.6206, 2.8225) knots 0 0 0 0 1 1 1 1
  spline S324 degree 3 poles (-74.6206, 2.8225) (-75.0741, 3.7296) (-75.5754, 4.3741) (-75.8141, 4.3741) knots 0 0 0 0 1 1 1 1
  spline S325 degree 3 poles (-75.8141, 4.3741) (-76.1483, 4.3741) (-76.5303, 3.479) (-76.5303, 2.7032) knots 0 0 0 0 1 1 1 1
  spline S326 degree 3 poles (-76.5303, 2.7032) (-76.5303, 2.2496) (-76.4348, 1.8558) (-76.1603, 1.2829) knots 0 0 0 0 1 1 1 1
  spline S327 degree 3 poles (-76.1603, 1.2829) (-75.647, 0.1848) (-74.2506, -2.1426) (-73.248, -3.5629) knots 0 0 0 0 1 1 1 1
  spline S328 degree 3 poles (-73.248, -3.5629) (-71.6487, -5.8545) (-71.3622, -6.0813) (-70.849, -5.5203) knots 0 0 0 0 1 1 1 1
  spline S329 degree 3 poles (-58.6152, -1.9039) (-57.3023, -1.6413) (-55.9656, -1.14) (-53.2562, 0.1013) knots 0 0 0 0 1 1 1 1
  spline S330 degree 3 poles (-53.2562, 0.1013) (-52.8266, 0.3042) (-51.9672, 0.6861) (-51.3466, 0.9725) knots 0 0 0 0 1 1 1 1
  spline S331 degree 3 poles (-51.3466, 0.9725) (-47.933, 2.5122) (-40.6405, 6.2122) (-36.487, 8.5276) knots 0 0 0 0 1 1 1 1
  spline S332 degree 3 poles (-36.487, 8.5276) (-34.5415, 9.6018) (-33.3241, 10.306) (-28.8842, 12.9318) knots 0 0 0 0 1 1 1 1
  spline S333 degree 3 poles (-28.8842, 12.9318) (-26.1032, 14.567) (-24.2532, 16.3095) (-23.3103, 18.1834) knots 0 0 0 0 1 1 1 1
  spline S334 degree 3 poles (-23.3103, 18.1834) (-23.0358, 18.7324) (-22.9881, 19.556) (-23.191, 20.093) knots 0 0 0 0 1 1 1 1
  spline S335 degree 3 poles (-23.191, 20.093) (-23.6087, 21.215) (-25.6377, 22.2414) (-27.9771, 22.504) knots 0 0 0 0 1 1 1 1
  spline S336 degree 3 poles (-27.9771, 22.504) (-31.3309, 22.8859) (-55.4762, 23.2917) (-57.0875, 22.9934) knots 0 0 0 0 1 1 1 1
  spline S337 degree 3 poles (-57.0875, 22.9934) (-58.5078, 22.7308) (-60.2981, 21.7521) (-61.062, 20.7972) knots 0 0 0 0 1 1 1 1
  spline S338 degree 3 poles (-61.062, 20.7972) (-62.1004, 19.544) (-62.5658, 18.4579) (-63.1507, 15.8918) knots 0 0 0 0 1 1 1 1
  spline S339 degree 3 poles (-63.1507, 15.8918) (-64.1652, 11.416) (-64.38, 10.0554) (-64.8933, 4.9112) knots 0 0 0 0 1 1 1 1
  spline S340 degree 3 poles (-64.8933, 4.9112) (-65.0245, 3.5506) (-64.9649, 1.4738) (-64.7858, 0.9009) knots 0 0 0 0 1 1 1 1
  spline S341 degree 3 poles (-64.7858, 0.9009) (-64.4158, -0.2807) (-63.3775, -1.4265) (-62.3152, -1.7965) knots 0 0 0 0 1 1 1 1
  spline S342 degree 3 poles (-62.3152, -1.7965) (-62.0049, -1.9158) (-61.7662, -2.0352) (-61.79, -2.071) knots 0 0 0 0 1 1 1 1
  spline S343 degree 3 poles (-61.79, -2.071) (-61.9213, -2.2739) (-59.8923, -2.1665) (-58.6152, -1.9039) knots 0 0 0 0 1 1 1 1
  spline S344 degree 3 poles (-68.3187, 0.2564) (-68.0681, 0.8054) (-68.1516, 1.438) (-68.5694, 2.2496) knots 0 0 0 0 1 1 1 1
  spline S345 degree 3 poles (-68.5694, 2.2496) (-69.751, 4.4815) (-71.2787, 7.6086) (-71.9232, 9.1483) knots 0 0 0 0 1 1 1 1
  spline S346 degree 3 poles (-71.9232, 9.1483) (-72.1022, 9.578) (-72.3051, 10.0076) (-72.3529, 10.1151) knots 0 0 0 0 1 1 1 1
  spline S347 degree 3 poles (-72.3529, 10.1151) (-72.4364, 10.2702) (-73.1287, 12.0128) (-73.9283, 14.0657) knots 0 0 0 0 1 1 1 1
  spline S348 degree 3 poles (-73.9283, 14.0657) (-74.2267, 14.8295) (-74.7041, 14.7818) (-75.1219, 13.9463) knots 0 0 0 0 1 1 1 1
  spline S349 degree 3 poles (-75.1219, 13.9463) (-75.3367, 13.4928) (-75.3964, 13.1944) (-75.3964, 12.3708) knots 0 0 0 0 1 1 1 1
  spline S350 degree 3 poles (-75.3964, 12.3708) (-75.3845, 11.4279) (-75.3487, 11.2609) (-74.8593, 10.1628) knots 0 0 0 0 1 1 1 1
  spline S351 degree 3 poles (-74.8593, 10.1628) (-73.8925, 7.9786) (-71.6726, 3.7177) (-70.9206, 2.5838) knots 0 0 0 0 1 1 1 1
  spline S352 degree 3 poles (-70.9206, 2.5838) (-70.8132, 2.4167) (-70.4671, 1.8916) (-70.1568, 1.4141) knots 0 0 0 0 1 1 1 1
  spline S353 degree 3 poles (-70.1568, 1.4141) (-69.8584, 0.9487) (-69.4884, 0.4235) (-69.3452, 0.2564) knots 0 0 0 0 1 1 1 1
  spline S354 degree 3 poles (-69.3452, 0.2564) (-68.999, -0.1494) (-68.4977, -0.1375) (-68.3187, 0.2564) knots 0 0 0 0 1 1 1 1
  spline S355 degree 3 poles (-25.0648, 7.2864) (-24.3607, 7.6579) (-24.6148, 7.6472) (-24.3964, 7.8354) knots 0 0 0 0 1 1 1 1
  spline S356 degree 3 poles (-24.3964, 7.8354) (-23.6774, 8.4551) (-22.451, 9.4228) (-22.2839, 9.7451) knots 0 0 0 0 1 1 1 1
  spline S357 degree 3 poles (-22.2839, 9.7451) (-22.0332, 10.2344) (-22.0571, 11.1534) (-22.3316, 11.607) knots 0 0 0 0 1 1 1 1
  spline S358 degree 3 poles (-22.3316, 11.607) (-22.8687, 12.4902) (-24.0622, 12.7647) (-25.1006, 12.2634) knots 0 0 0 0 1 1 1 1
  spline S359 degree 3 poles (-25.1006, 12.2634) (-28.0725, 10.8073) (-28.6693, 10.2822) (-28.6693, 9.0647) knots 0 0 0 0 1 1 1 1
  spline S360 degree 3 poles (-28.6693, 9.0647) (-28.6693, 7.0715) (-26.8257, 6.3571) (-25.0648, 7.2864) knots 0 0 0 0 1 1 1 1
  spline S361 degree 3 poles (-67.6623, 9.387) (-67.1132, 9.8167) (-67.1252, 10.2822) (-67.7339, 11.9889) knots 0 0 0 0 1 1 1 1
  spline S362 degree 3 poles (-67.7339, 11.9889) (-68.9632, 15.4502) (-70.2881, 19.7589) (-70.9803, 22.5756) knots 0 0 0 0 1 1 1 1
  spline S363 degree 3 poles (-70.9803, 22.5756) (-71.1593, 23.3275) (-71.398, 23.984) (-71.5293, 24.1272) knots 0 0 0 0 1 1 1 1
  spline S364 degree 3 poles (-71.5293, 24.1272) (-71.8874, 24.4972) (-72.329, 24.2585) (-72.7467, 23.4708) knots 0 0 0 0 1 1 1 1
  spline S365 degree 3 poles (-72.7467, 23.4708) (-73.069, 22.874) (-73.0929, 22.7427) (-73.0213, 21.9788) knots 0 0 0 0 1 1 1 1
  spline S366 degree 3 poles (-73.0213, 21.9788) (-72.9019, 20.5585) (-71.2429, 15.4382) (-69.8822, 12.3112) knots 0 0 0 0 1 1 1 1
  spline S367 degree 3 poles (-69.8822, 12.3112) (-68.82, 9.8644) (-68.4142, 9.1722) (-68.0442, 9.1483) knots 0 0 0 0 1 1 1 1
  spline S368 degree 3 poles (-68.0442, 9.1483) (-67.9965, 9.1483) (-67.8294, 9.2557) (-67.6623, 9.387) knots 0 0 0 0 1 1 1 1
  spline S369 degree 3 poles (-15.1942, 11.595) (-14.4543, 12.2873) (-14.1797, 12.9796) (-14.2633, 13.9224) knots 0 0 0 0 1 1 1 1